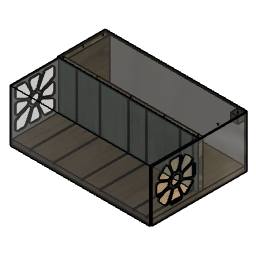
ionenantrieb v2 v2 (Autodesk Fusion 360 design; units mm, degrees)
Autodesk Fusion 360 part; units mm, degrees
sketch "Skizze1" plane through (0, 0, 0) normal (0, 0, 1) x (1, 0, 0)
  line L0 (0, 0) -> (300, 0)
  line L1 (300, 0) -> (300, 200)
  line L2 (300, 200) -> (0, 200)
  line L3 (0, 200) -> (0, 0)
  dimension "d1" = 300
  dimension "d2" = 200
  constraint horizontal L0
  constraint vertical L1
  constraint horizontal L2
  constraint vertical L3
  constraint coincident L0.start L3.end
  measures "d1" distance of L0.start L0.end
  measures "d2" distance of L0.start L2.end
extrude "Extrusion1" add sketch "Skizze1" along normal blind 10 makes body 1
sketch "Skizze2" plane through (0, 0, 10) normal (0, 0, 1) x (-1, 0, 0)
  line L0 (0, -200) -> (0, 0)
  line L1 (0, 0) -> (-300, 0)
  line L2 (-300, 0) -> (-300, -200)
  line L3 (-300, -200) -> (0, -200)
  line L4 (0, -100) -> (-300, -100)
  line L5 (-300, -100) -> (-300, -110)
  line L6 (-300, -110) -> (0, -110)
  line L7 (0, -110) -> (0, -100)
  constraint horizontal L4
  constraint vertical L5
  constraint horizontal L6
  constraint vertical L7
  constraint coincident L2 L5.end
  constraint midpoint L0 L4.start
extrude "Extrusion1'" add sketch "Skizze2" along normal blind 100 separate body contours L0 L2 L4 L5 L6 L7 makes body 2 in component "Component"
sketch "Skizze3" plane through (0, 200, 0) normal (0, 1, 0) x (-1, 0, 0)
  line L0 (-300, 0) -> (0, 0)
  line L1 (0, 0) -> (0, 10)
  line L2 (0, 10) -> (-300, 10)
  line L3 (-300, 10) -> (-300, 0)
  line L4 (-300, 0) -> (0, 0)
  line L5 (0, 0) -> (0, 110)
  line L6 (0, 110) -> (-300, 110)
  line L7 (-300, 110) -> (-300, 0)
  constraint horizontal L4
  constraint vertical L5
  constraint horizontal L6
  constraint vertical L7
  constraint coincident L0.start L3.end
extrude "Extrusion1''" add sketch "Skizze3" along normal blind 2.5 separate body makes body 3 in component "Component'"
sketch "Skizze4" plane through (0, 202.5, 0) normal (0, 1, 0) x (-1, 0, 0)
  line L0 (-300, 110) -> (-300, 0)
  line L1 (-300, 0) -> (0, 0)
  line L2 (0, 0) -> (0, 110)
  line L3 (0, 110) -> (-300, 110)
  circle A0 centre (-290, 5) radius 1
  circle A1 centre (-220, 5) radius 1
  circle A2 centre (-150, 5) radius 1
  circle A3 centre (-80, 5) radius 1
  circle A4 centre (-10, 5) radius 1
  dimension "d9" = 2
  dimension "d12" = 280
  dimension "d13" = 0
  measures "d9" diameter of A0
extrude "Extrusion2" cut sketch "Skizze4" against normal blind 2.5 contours A0 | A1 | A2 | A3 | A4 bodies 3 in component "Component'"
sketch "Skizze5" plane through (300, 0, 0) normal (1, 0, 0) x (0, 1, 0)
  line L0 (0, 0) -> (200, 0)
  line L1 (200, 0) -> (200, 10)
  line L2 (200, 10) -> (0, 10)
  line L3 (0, 10) -> (0, 0)
  line L4 (202.5, 0) -> (-1.5, 0)
  line L5 (-1.5, 0) -> (-1.5, 110)
  line L6 (-1.5, 110) -> (202.5, 110)
  line L7 (202.5, 110) -> (202.5, 0)
  dimension "d16" = 204
  constraint horizontal L4
  constraint vertical L5
  constraint horizontal L6
  constraint vertical L7
  measures "d16" distance of L4.start L4.end
extrude "Extrusion1'''" add sketch "Skizze5" along normal blind 2.5 separate body makes body 4 in component "Component''"
sketch "Skizze6" plane through (302.5, 0, 0) normal (1, 0, 0) x (0, 1, 0)
  line L0 (202.5, 110) -> (-1.5, 110)
  line L1 (-1.5, 110) -> (-1.5, 0)
  line L2 (-1.5, 0) -> (202.5, 0)
  line L3 (202.5, 0) -> (202.5, 110)
  circle A0 centre (10, 5) radius 1
  circle A1 centre (105, 5) radius 1
  line L4 (10, 5) -> (105, 5)
  circle A2 centre (57.5, 5) radius 1
  circle A3 centre (147.5, 5) radius 1
  circle A4 centre (190, 5) radius 1
  circle A5 centre (105, 52.5) radius 1
  circle A6 centre (105, 100) radius 1
  dimension "d19" = 2
  dimension "d20" = 2
  dimension "d21" = 2
  dimension "d24" = 85
  dimension "d25" = 0
  dimension "d28" = 0
  dimension "d29" = 95
  constraint coincident A0.centre L4.start
  constraint coincident A1.centre L4.end
  constraint midpoint L4 A2.centre
  measures "d19" diameter of A0
  measures "d20" diameter of A1
  measures "d21" diameter of A2
sketch "Skizze7" plane through (0, 0, 0) normal (-1, 0, 0) x (0, -1, 0)
  line L0 (-200, 0) -> (0, 0)
  line L1 (0, 0) -> (0, 10)
  line L2 (0, 10) -> (-200, 10)
  line L3 (-200, 10) -> (-200, 0)
  line L4 (-110, 110) -> (-200, 110)
  line L5 (-200, 110) -> (-200, 10)
  line L6 (-200, 10) -> (-110, 10)
  line L7 (-110, 10) -> (-110, 110)
  constraint horizontal L4
  constraint vertical L5
  constraint horizontal L6
  constraint vertical L7
  constraint coincident L2.end L3.start
extrude "Extrusion1''''" add sketch "Skizze7" against normal blind 10 separate body contours L2 L4 L5 L6 L7 makes body 5 in component "Component'''"
sketch "Skizze8" plane through (0, 0, 0) normal (-1, 0, 0) x (0, -1, 0)
  line L0 (-110, 10) -> (-100, 10)
  line L1 (-100, 10) -> (-100, 110)
  line L2 (-100, 110) -> (-110, 110)
  line L3 (-110, 110) -> (-110, 10)
  line L4 (-202.5, 0) -> (1.5, 0)
  line L5 (1.5, 0) -> (1.5, 110)
  line L6 (1.5, 110) -> (-202.5, 110)
  line L7 (-202.5, 110) -> (-202.5, 0)
  constraint horizontal L4
  constraint vertical L5
  constraint horizontal L6
  constraint vertical L7
extrude "Extrusion1'''''" add sketch "Skizze8" along normal blind 2.5 separate body makes body 6 in component "Component''''"
ref_plane "Arbeitsebene1" through (150, 100.5, 55) normal (1, 0, 0) x (0, 1, 0)
sketch "Skizze9" plane through (-2.5, 0, 0) normal (-1, 0, 0) x (0, -1, 0)
  line L0 (-202.5, 110) -> (-202.5, 0)
  line L1 (-202.5, 0) -> (1.5, 0)
  line L2 (1.5, 0) -> (1.5, 110)
  line L3 (1.5, 110) -> (-202.5, 110)
  circle A0 centre (-190, 5) radius 1
  circle A1 centre (-10, 5) radius 1
  circle A2 centre (-105, 5) radius 1
  circle A3 centre (-150, 5) radius 1
  circle A4 centre (-57.5, 5) radius 1
  circle A5 centre (-105, 52.5) radius 1
  circle A6 centre (-105, 100) radius 1
  dimension "d34" = 2
  dimension "d35" = 2
  dimension "d36" = 2
  dimension "d37" = 2
  dimension "d38" = 2
  dimension "d41" = 0
  dimension "d42" = 95
  measures "d34" diameter of A0
  measures "d35" diameter of A1
  measures "d36" diameter of A2
  measures "d37" diameter of A3
  measures "d38" diameter of A4
extrude "Extrusion2'" cut sketch "Skizze9" against normal blind 2.5 contours A0 | A1 | A2 | A3 | A4 | A5 | A6 bodies 6 in component "Component''''"
sketch "Skizze10" plane through (0, 0, 110) normal (0, 0, 1) x (-1, 0, 0)
  line L0 (0, -110) -> (0, -100)
  line L1 (0, -100) -> (-300, -100)
  line L2 (-300, -100) -> (-300, -110)
  line L3 (-300, -110) -> (0, -110)
  line L4 (-302.5, -202.5) -> (2.5, -202.5)
  line L5 (2.5, -202.5) -> (2.5, -100)
  line L6 (2.5, -100) -> (-302.5, -100)
  line L7 (-302.5, -100) -> (-302.5, -202.5)
  constraint horizontal L4
  constraint vertical L5
  constraint horizontal L6
  constraint vertical L7
extrude "Extrusion1''''''" add sketch "Skizze10" along normal blind 2.5 separate body makes body 7 in component "Component'''''"
sketch "Skizze11" plane through (0, 0, 112.5) normal (0, 0, 1) x (-1, 0, 0)
  line L0 (-302.5, -100) -> (-302.5, -202.5)
  line L1 (-302.5, -202.5) -> (2.5, -202.5)
  line L2 (2.5, -202.5) -> (2.5, -100)
  line L3 (2.5, -100) -> (-302.5, -100)
  circle A0 centre (-295, -105) radius 1
  circle A1 centre (-222.5, -105) radius 1
  circle A2 centre (-150, -105) radius 1
  circle A3 centre (-77.5, -105) radius 1
  circle A4 centre (-5, -105) radius 1
  circle A5 centre (-5, -190) radius 1
  line L4 (-5, -190) -> (-5, -105)
  circle A6 centre (-5, -147.5) radius 1
  line L5 (-150, -105) -> (-150, -112.2245)
  circle A7 centre (-295, -147.5) radius 1
  circle A8 centre (-295, -190) radius 1
  point P0 (-295, -190)
  dimension "d47" = 2
  dimension "d50" = 290
  dimension "d51" = 0
  dimension "d52" = 2
  dimension "d53" = 2
  constraint coincident A5.centre L4.start
  constraint coincident A4.centre L4.end
  constraint perpendicular L3 L4
  constraint midpoint L4 A6.centre
  constraint coincident A2.centre L5.start
  constraint vertical L5
  constraint symmetric A5 L5 A8
  constraint symmetric A5.centre L5 P0
  constraint symmetric A6 L5 A7
  measures "d47" diameter of A0
  measures "d52" diameter of A5
  measures "d53" diameter of A6
extrude "Extrusion2''" cut sketch "Skizze11" against normal blind 2.5 contours A0 | A1 | A2 | A3 | A4 | A5 | L4 A6 | L4 A6 | A7 | A8 bodies 7 in component "Component'''''"
sketch "Skizze12" plane through (0, 200, 0) normal (0, -1, 0) x (1, 0, 0)
  circle A0 centre (80, 5) radius 1
  circle A1 centre (290, 5) radius 1
  circle A2 centre (220, 5) radius 1
  circle A3 centre (150, 5) radius 1
  circle A4 centre (10, 5) radius 1
  line L0 (300, 0) -> (300, 110)
  line L1 (300, 110) -> (0, 110)
  line L2 (0, 110) -> (0, 0)
  line L3 (0, 0) -> (300, 0)
  line L4 (300, 110) -> (285, 110)
  line L5 (285, 110) -> (285, 95)
  line L6 (285, 95) -> (300, 95)
  line L7 (300, 95) -> (300, 110)
  constraint horizontal L4
  constraint vertical L5
  constraint horizontal L6
  constraint vertical L7
  constraint coincident L0.end L1.start
extrude "Extrusion1'''''''" add sketch "Skizze12" along normal blind 15 separate body contours L0 L1 L4 L5 L6 L7 makes body 8 in component "Component''''''"
sketch "Skizze13" plane through (302.5, 0, 0) normal (1, 0, 0) x (0, 1, 0)
  line L0 (202.5, 110) -> (-1.5, 110)
  line L1 (-1.5, 110) -> (-1.5, 0)
  line L2 (-1.5, 0) -> (202.5, 0)
  line L3 (202.5, 0) -> (202.5, 110)
  line L4 (100, 10) -> (0, 10)
  line L5 (0, 10) -> (0, 110)
  line L6 (0, 110) -> (100, 110)
  line L7 (100, 110) -> (100, 10)
  circle A0 centre (50, 60) radius 10
  line L8 (92, 18) -> (8, 18)
  line L9 (8, 18) -> (8, 102)
  line L10 (41.854, 102) -> (58.146, 102)
  line L11 (92, 102) -> (92, 18)
  arc A1 (51.1575, 73.9521) -> (48.8425, 73.9521) centre (50, 60) ccw
  line L12 (50, 60) -> (50, 70)
  line L13 (50, 60) -> (46.5798, 69.3969)
  line L14 (43.7307, 77.2249) -> (37.1555, 95.2899)
  line L15 (50, 60) -> (53.4202, 69.3969)
  line L16 (56.2693, 77.2249) -> (62.8445, 95.2899)
  arc A2 (41.854, 102) -> (37.1555, 95.2899) centre (41.854, 97) ccw
  arc A3 (62.8445, 95.2899) -> (58.146, 102) centre (58.146, 97) ccw
  arc A4 (43.7307, 77.2249) -> (48.8425, 73.9521) centre (48.4291, 78.935) ccw
  arc A5 (51.1575, 73.9521) -> (56.2693, 77.2249) centre (51.5709, 78.935) ccw
  line L17 (14.5414, 83.9384) -> (26.0616, 95.4586)
  arc A6 (33.3871, 67.7467) -> (39.3159, 69.0471) centre (35.5002, 72.2783) ccw
  line L18 (42.2533, 76.6129) -> (34.1287, 94.0361)
  arc A7 (14.5414, 83.9384) -> (15.9639, 75.8713) centre (18.077, 80.4029) ccw
  arc A8 (40.9529, 70.6841) -> (39.3159, 69.0471) centre (50, 60) ccw
  line L19 (33.3871, 67.7467) -> (15.9639, 75.8713)
  arc A9 (40.9529, 70.6841) -> (42.2533, 76.6129) centre (37.7217, 74.4998) ccw
  arc A10 (34.1287, 94.0361) -> (26.0616, 95.4586) centre (29.5971, 91.923) ccw
  line L20 (8, 51.854) -> (8, 68.146)
  arc A11 (32.7752, 53.7307) -> (36.0479, 58.8425) centre (31.065, 58.4291) ccw
  line L21 (32.7752, 66.2693) -> (14.7101, 72.8445)
  arc A12 (8, 51.854) -> (14.7101, 47.1555) centre (13, 51.854) ccw
  arc A13 (36.0479, 61.1575) -> (36.0479, 58.8425) centre (50, 60) ccw
  line L22 (32.7752, 53.7307) -> (14.7101, 47.1555)
  arc A14 (36.0479, 61.1575) -> (32.7752, 66.2693) centre (31.065, 61.5709) ccw
  arc A15 (14.7101, 72.8445) -> (8, 68.146) centre (13, 68.146) ccw
  line L23 (26.0616, 24.5414) -> (14.5414, 36.0616)
  arc A16 (42.2533, 43.3871) -> (40.9529, 49.3159) centre (37.7217, 45.5002) ccw
  line L24 (33.3871, 52.2533) -> (15.9639, 44.1287)
  arc A17 (26.0616, 24.5414) -> (34.1287, 25.9639) centre (29.5971, 28.077) ccw
  arc A18 (39.3159, 50.9529) -> (40.9529, 49.3159) centre (50, 60) ccw
  line L25 (42.2533, 43.3871) -> (34.1287, 25.9639)
  arc A19 (39.3159, 50.9529) -> (33.3871, 52.2533) centre (35.5002, 47.7217) ccw
  arc A20 (15.9639, 44.1287) -> (14.5414, 36.0616) centre (18.077, 39.5971) ccw
  line L26 (58.146, 18) -> (41.854, 18)
  arc A21 (56.2693, 42.7751) -> (51.1575, 46.0479) centre (51.5709, 41.065) ccw
  line L27 (43.7307, 42.7751) -> (37.1555, 24.7101)
  arc A22 (58.146, 18) -> (62.8445, 24.7101) centre (58.146, 23) ccw
  arc A23 (48.8425, 46.0479) -> (51.1575, 46.0479) centre (50, 60) ccw
  line L28 (56.2693, 42.7751) -> (62.8445, 24.7101)
  arc A24 (48.8425, 46.0479) -> (43.7307, 42.7751) centre (48.4291, 41.065) ccw
  arc A25 (37.1555, 24.7101) -> (41.854, 18) centre (41.854, 23) ccw
  line L29 (85.4586, 36.0616) -> (73.9384, 24.5414)
  arc A26 (66.6129, 52.2533) -> (60.6841, 50.9529) centre (64.4998, 47.7217) ccw
  line L30 (57.7467, 43.3871) -> (65.8713, 25.9639)
  arc A27 (85.4586, 36.0616) -> (84.0361, 44.1287) centre (81.9231, 39.5971) ccw
  arc A28 (59.0471, 49.3159) -> (60.6841, 50.9529) centre (50, 60) ccw
  line L31 (66.6129, 52.2533) -> (84.0361, 44.1287)
  arc A29 (59.0471, 49.3159) -> (57.7467, 43.3871) centre (62.2783, 45.5002) ccw
  arc A30 (65.8713, 25.9639) -> (73.9384, 24.5414) centre (70.4029, 28.077) ccw
  line L32 (92, 68.146) -> (92, 51.854)
  arc A31 (67.2249, 66.2693) -> (63.9521, 61.1575) centre (68.935, 61.5709) ccw
  line L33 (67.2249, 53.7307) -> (85.2899, 47.1555)
  arc A32 (92, 68.146) -> (85.2899, 72.8445) centre (87, 68.146) ccw
  arc A33 (63.9521, 58.8425) -> (63.9521, 61.1575) centre (50, 60) ccw
  line L34 (67.2249, 66.2693) -> (85.2899, 72.8445)
  arc A34 (63.9521, 58.8425) -> (67.2249, 53.7307) centre (68.935, 58.4291) ccw
  arc A35 (85.2899, 47.1555) -> (92, 51.854) centre (87, 51.854) ccw
  line L35 (73.9384, 95.4586) -> (85.4586, 83.9384)
  arc A36 (57.7467, 76.6129) -> (59.0471, 70.6841) centre (62.2783, 74.4998) ccw
  line L36 (66.6129, 67.7467) -> (84.0361, 75.8713)
  arc A37 (73.9384, 95.4586) -> (65.8713, 94.0361) centre (70.4029, 91.923) ccw
  arc A38 (60.6841, 69.0471) -> (59.0471, 70.6841) centre (50, 60) ccw
  line L37 (57.7467, 76.6129) -> (65.8713, 94.0361)
  arc A39 (60.6841, 69.0471) -> (66.6129, 67.7467) centre (64.4998, 72.2783) ccw
  arc A40 (84.0361, 75.8713) -> (85.4586, 83.9384) centre (81.9231, 80.4029) ccw
  dimension "d58" = 20
  dimension "d61" = 20
  dimension "d62" = 20
  dimension "d63" = 5
  dimension "d64" = 5
  dimension "d66" = 360
  constraint horizontal L4
  constraint vertical L5
  constraint horizontal L6
  constraint vertical L7
  constraint coincident L0 L5.end
  constraint coincident A0.centre A1.centre
  constraint perpendicular L10 L12
  constraint concentric A0 A1
  constraint coincident A0 L12.end
  constraint coincident A0 L13.end
  constraint collinear L13 L14
  constraint coincident A0 L15.end
  constraint collinear L15 L16
  constraint parallel L4 L8
  constraint parallel L5 L9
  constraint parallel L6 L10
  constraint parallel L7 L11
  constraint tangent L14 A2
  constraint tangent L10 A2
  constraint tangent L16 A3
  constraint tangent L10 A3
  constraint equal A2 A3
  constraint tangent L14 A4
  constraint tangent A1 A4
  constraint tangent L16 A5
  constraint tangent A1 A5
  constraint equal A4 A5
  measures "d58" diameter of A0
  measures "d61" angle of L12 L15
  measures "d62" angle of L12 L13
  measures "d63" radius of A2
  measures "d64" radius of A4
extrude "Extrusion2'''" cut sketch "Skizze13" against normal blind 5 contours A0 L13 L15 | A0 L12 L15 | A0 L12 L13 | L8 L26 A21 L27 A22 A23 L28 A24 A25 | L9 L20 A11 L21 A12 A13 L22 A14 A15 | L10 A1 L14 L16 A2 A3 A4 A5 | L11 L32 A31 L33 A32 A33 L34 A34 A35 | L17 A6 L18 A7 A8 L19 A9 A10 | L23 A16 L24 A17 A18 L25 A19 A20 | L29 A26 L30 A27 A28 L31 A29 A30 | L35 A36 L36 A37 A38 L37 A39 A40 bodies 4 in component "Component''"
sketch "Skizze14" plane through (-2.5, 0, 0) normal (-1, 0, 0) x (0, -1, 0)
  circle A0 centre (-105, 100) radius 1
  circle A1 centre (-57.5, 5) radius 1
  circle A2 centre (-105, 5) radius 1
  circle A3 centre (-10, 5) radius 1
  circle A4 centre (-190, 5) radius 1
  circle A5 centre (-105, 52.5) radius 1
  circle A6 centre (-150, 5) radius 1
  line L0 (-202.5, 110) -> (-202.5, 0)
  line L1 (-202.5, 0) -> (1.5, 0)
  line L2 (1.5, 0) -> (1.5, 110)
  line L3 (1.5, 110) -> (-202.5, 110)
  line L4 (-100, 110) -> (0, 110)
  line L5 (0, 110) -> (0, 10)
  line L6 (0, 10) -> (-100, 10)
  line L7 (-100, 10) -> (-100, 110)
  circle A7 centre (-50, 60) radius 10
  line L8 (-50, 70) -> (-50, 74)
  line L9 (-92, 60) -> (-92, 67.452)
  line L10 (-92, 83.6091) -> (-92, 97)
  line L11 (-66.4752, 68.0355) -> (-89.1919, 79.1151)
  line L12 (-67.3316, 65.9678) -> (-85.3722, 72.1796)
  line L13 (-33.5248, 68.0355) -> (-10.8081, 79.1151)
  line L14 (-32.6684, 65.9678) -> (-14.6278, 72.1796)
  line L15 (-44.0322, 77.3316) -> (-37.8204, 95.3722)
  line L16 (-41.9645, 76.4752) -> (-30.8849, 99.1919)
  line L17 (-55.9678, 77.3316) -> (-62.1796, 95.3722)
  line L18 (-58.0355, 76.4752) -> (-69.1151, 99.1919)
  line L19 (-87, 102) -> (-73.6091, 102)
  line L20 (-57.452, 102) -> (-42.548, 102)
  line L21 (-26.3909, 102) -> (-13, 102)
  line L22 (-8, 97) -> (-8, 83.6091)
  line L23 (-8, 67.452) -> (-8, 60)
  arc A8 (-87, 102) -> (-92, 97) centre (-87, 97) ccw
  arc A9 (-57.452, 102) -> (-62.1796, 95.3722) centre (-57.452, 97) ccw
  arc A10 (-37.8204, 95.3722) -> (-42.548, 102) centre (-42.548, 97) ccw
  arc A11 (-8, 97) -> (-13, 102) centre (-13, 97) ccw
  arc A12 (-69.1151, 99.1919) -> (-73.6091, 102) centre (-73.6091, 97) ccw
  arc A13 (-92, 83.6091) -> (-89.1919, 79.1151) centre (-87, 83.6091) ccw
  arc A14 (-26.3909, 102) -> (-30.8849, 99.1919) centre (-26.3909, 97) ccw
  arc A15 (-10.8081, 79.1151) -> (-8, 83.6091) centre (-13, 83.6091) ccw
  arc A16 (-8, 67.452) -> (-14.6278, 72.1796) centre (-13, 67.452) ccw
  arc A17 (-85.3722, 72.1796) -> (-92, 67.452) centre (-87, 67.452) ccw
  arc A18 (-59.2322, 70.5245) -> (-60.5245, 69.2322) centre (-50, 60) ccw
  arc A19 (-49.0862, 73.9701) -> (-50.9138, 73.9701) centre (-50, 60) ccw
  arc A20 (-63.9701, 60.9138) -> (-36.0299, 60.9138) centre (-50, 60) ccw
  arc A21 (-39.4755, 69.2322) -> (-40.7678, 70.5245) centre (-50, 60) ccw
  arc A22 (-66.4752, 68.0355) -> (-60.5245, 69.2322) centre (-64.2833, 72.5294) ccw
  arc A23 (-59.2322, 70.5245) -> (-58.0355, 76.4752) centre (-62.5294, 74.2833) ccw
  arc A24 (-55.9678, 77.3316) -> (-50.9138, 73.9701) centre (-51.2402, 78.9595) ccw
  arc A25 (-49.0862, 73.9701) -> (-44.0322, 77.3316) centre (-48.7598, 78.9595) ccw
  arc A26 (-41.9645, 76.4752) -> (-40.7678, 70.5245) centre (-37.4706, 74.2833) ccw
  arc A27 (-39.4755, 69.2322) -> (-33.5248, 68.0355) centre (-35.7167, 72.5294) ccw
  arc A28 (-63.9701, 60.9138) -> (-67.3316, 65.9678) centre (-68.9595, 61.2402) ccw
  arc A29 (-32.6684, 65.9678) -> (-36.0299, 60.9138) centre (-31.0405, 61.2402) ccw
  line L24 (-92, 60) -> (-85, 60)
  arc A30 (-92, 23) -> (-87, 18) centre (-87, 23) ccw
  arc A31 (-62.1796, 24.6278) -> (-57.452, 18) centre (-57.452, 23) ccw
  line L25 (-66.4752, 51.9645) -> (-89.1919, 40.8849)
  line L26 (-92, 36.3909) -> (-92, 23)
  arc A32 (-73.6091, 18) -> (-69.1151, 20.8081) centre (-73.6091, 23) ccw
  arc A33 (-60.5245, 50.7678) -> (-59.2322, 49.4755) centre (-50, 60) ccw
  arc A34 (-58.0355, 43.5248) -> (-59.2322, 49.4755) centre (-62.5294, 45.7167) ccw
  line L27 (-55.9678, 42.6684) -> (-62.1796, 24.6278)
  line L28 (-50, 50) -> (-50, 46)
  arc A35 (-92, 52.548) -> (-85.3722, 47.8204) centre (-87, 52.548) ccw
  line L29 (-87, 18) -> (-73.6091, 18)
  arc A36 (-50.9138, 46.0299) -> (-55.9678, 42.6684) centre (-51.2402, 41.0405) ccw
  line L30 (-67.3316, 54.0322) -> (-85.3722, 47.8204)
  arc A37 (-50.9138, 46.0299) -> (-49.0862, 46.0299) centre (-50, 60) ccw
  arc A38 (-89.1919, 40.8849) -> (-92, 36.3909) centre (-87, 36.3909) ccw
  line L31 (-58.0355, 43.5248) -> (-69.1151, 20.8081)
  arc A39 (-67.3316, 54.0322) -> (-63.9701, 59.0862) centre (-68.9595, 58.7598) ccw
  line L32 (-92, 60) -> (-92, 52.548)
  arc A40 (-33.5248, 51.9645) -> (-39.4755, 50.7678) centre (-35.7167, 47.4706) ccw
  arc A41 (-44.0322, 42.6684) -> (-49.0862, 46.0299) centre (-48.7598, 41.0405) ccw
  arc A42 (-14.6278, 47.8204) -> (-8, 52.548) centre (-13, 52.548) ccw
  line L33 (-32.6684, 54.0322) -> (-14.6278, 47.8204)
  line L34 (-26.3909, 18) -> (-13, 18)
  line L35 (-41.9645, 43.5248) -> (-30.8849, 20.8081)
  arc A43 (-40.7678, 49.4755) -> (-39.4755, 50.7678) centre (-50, 60) ccw
  line L36 (-57.452, 18) -> (-42.548, 18)
  line L37 (-8, 52.548) -> (-8, 60)
  arc A44 (-13, 18) -> (-8, 23) centre (-13, 23) ccw
  line L38 (-44.0322, 42.6684) -> (-37.8204, 24.6278)
  arc A45 (-36.0299, 59.0862) -> (-32.6684, 54.0322) centre (-31.0405, 58.7598) ccw
  arc A46 (-40.7678, 49.4755) -> (-41.9645, 43.5248) centre (-37.4706, 45.7167) ccw
  line L39 (-33.5248, 51.9645) -> (-10.8081, 40.8849)
  arc A47 (-42.548, 18) -> (-37.8204, 24.6278) centre (-42.548, 23) ccw
  line L40 (-8, 23) -> (-8, 36.3909)
  arc A48 (-8, 36.3909) -> (-10.8081, 40.8849) centre (-13, 36.3909) ccw
  arc A49 (-30.8849, 20.8081) -> (-26.3909, 18) centre (-26.3909, 23) ccw
  arc A50 (-60.5245, 50.7678) -> (-66.4752, 51.9645) centre (-64.2833, 47.4706) ccw
  point P0 (-50, 60)
  point P1 (-50, 60)
  dimension "d70" = 20
  dimension "d80" = 5
  dimension "d81" = 5
  dimension "d82" = 5
  dimension "d83" = 5
  constraint horizontal L4
  constraint vertical L5
  constraint horizontal L6
  constraint vertical L7
  constraint coincident L3 L4.start
  constraint parallel L7 L9
  constraint parallel L4 L19
  constraint parallel L5 L22
  constraint collinear L9 L10
  constraint coincident A7 L8.start
  constraint collinear L19 L20
  constraint collinear L20 L21
  constraint coincident L8.end A20
  constraint collinear L22 L23
  constraint coincident L23.end L22
  constraint tangent L19 A8
  constraint tangent L10 A8
  constraint tangent L20 A9
  constraint tangent L17 A9
  constraint equal A8 A9
  constraint tangent L15 A10
  constraint tangent L20 A10
  constraint equal A8 A10
  constraint tangent L21 A11
  constraint tangent L22 A11
  constraint equal A8 A11
  constraint tangent L18 A12
  constraint tangent L19 A12
  constraint equal A8 A12
  constraint tangent L11 A13
  constraint tangent L10 A13
  constraint equal A8 A13
  constraint tangent L16 A14
  constraint tangent L21 A14
  constraint equal A8 A14
  constraint tangent L13 A15
  constraint tangent L22 A15
  constraint equal A8 A15
  constraint tangent L14 A16
  constraint tangent L23 A16
  constraint equal A8 A16
  constraint tangent L12 A17
  constraint tangent L9 A17
  constraint equal A8 A17
  constraint concentric A7 A20
  constraint concentric A18 A20
  constraint concentric A19 A20
  constraint concentric A20 A21
  constraint tangent A18 A22
  constraint tangent L11 A22
  constraint tangent L18 A23
  constraint tangent A18 A23
  constraint equal A22 A23
  constraint tangent L17 A24
  constraint tangent A19 A24
  constraint equal A22 A24
  constraint tangent A19 A25
  constraint tangent L15 A25
  constraint equal A22 A25
  constraint tangent A21 A26
  constraint tangent L16 A26
  constraint equal A22 A26
  constraint tangent L13 A27
  constraint tangent A21 A27
  constraint equal A22 A27
  constraint tangent A20 A28
  constraint tangent L12 A28
  constraint tangent L14 A29
  constraint tangent A20 A29
  constraint perpendicular L9 L24
  constraint symmetric P1 L24 P0
  constraint symmetric L9.start L24 L32.start
  constraint symmetric L23.end L24 L37.end
  constraint symmetric L8.start L24 L28.start
  constraint symmetric L8.end L24 L28.end
  constraint symmetric L19.start L24 A30.end
  constraint symmetric L10.end L24 A30.start
  constraint symmetric A8 L24 A30
  constraint symmetric L20.start L24 A31.end
  constraint symmetric L17.end L24 A31.start
  constraint symmetric A9 L24 A31
  constraint symmetric L15.end L24 L38.end
  constraint symmetric L20.end L24 L36.end
  constraint symmetric A10 L24 A47
  constraint symmetric L21.end L24 L34.end
  constraint symmetric L22.start L24 A44.end
  constraint symmetric A11 L24 A44
  constraint symmetric L18.end L24 A32.end
  constraint symmetric L19.end L24 A32.start
  constraint symmetric A12 L24 A32
  constraint symmetric L11.end L24 L25.end
  constraint symmetric L10.start L24 L26.start
  constraint symmetric A13 L24 A38
  constraint symmetric L16.end L24 L35.end
  constraint symmetric L21.start L24 L34.start
  constraint symmetric A14 L24 A49
  constraint symmetric L13.end L24 L39.end
  constraint symmetric L22.end L24 L40.end
  constraint symmetric A15 L24 A48
  constraint symmetric L14.end L24 A42.start
  constraint symmetric L23.start L24 A42.end
  constraint symmetric A16 L24 A42
  constraint symmetric L12.end L24 A35.end
  constraint symmetric L9.end L24 A35.start
  constraint symmetric A17 L24 A35
  constraint symmetric A18 L24 A33
  constraint symmetric A19 L24 A37
  constraint symmetric A21 L24 A43
  constraint symmetric L11.start L24 L25.start
  constraint symmetric A18.end L24 A33.start
  constraint symmetric A22 L24 A50
  constraint symmetric L18.start L24 A34.start
  constraint symmetric A18.start L24 A33.end
  constraint symmetric A23 L24 A34
  constraint symmetric L17.start L24 L27.start
  constraint symmetric A19.end L24 A36.start
  constraint symmetric A24 L24 A36
  constraint symmetric L15.start L24 A41.start
  constraint symmetric A19.start L24 A37.end
  constraint symmetric A25 L24 A41
  constraint symmetric L16.start L24 L35.start
  constraint symmetric A21.end L24 A43.start
  constraint symmetric A26 L24 A46
  constraint symmetric L13.start L24 A40.start
  constraint symmetric A21.start L24 A40.end
  constraint symmetric A27 L24 A40
  constraint symmetric L12.start L24 L30.start
  constraint symmetric A20.start L24 A39.end
  constraint symmetric A28 L24 A39
  constraint symmetric L14.start L24 L33.start
  constraint symmetric A20.end L24 A45.start
  constraint symmetric A29 L24 A45
  measures "d70" diameter of A7
  measures "d80" radius of A8
  measures "d81" radius of A22
  measures "d82" radius of A28
  measures "d83" radius of A29
extrude "Extrusion3" cut sketch "Skizze14" against normal blind 2.5 contours A7 | L9 L12 A17 A20 A28 A35 L30 A39 L32 | L10 L11 L18 L19 A8 A12 A13 A18 A22 A23 | L13 L16 L21 L22 A11 A14 A15 A21 A26 A27 | L14 L23 A16 A20 A29 A42 L33 L37 A45 | L15 L17 L20 A9 A10 A19 A24 A25 | A20 A30 L25 L26 A32 A33 A34 L29 A38 L31 A50 | A20 A31 L27 A36 A37 A41 L36 L38 A47 | A20 A40 L34 L35 A43 A44 A46 L39 L40 A48 A49 bodies 6 in component "Component''''"
sketch "Skizze15" plane through (0, 0, 10) normal (0, 0, 1) x (-1, 0, 0)
  line L0 (0, -200) -> (0, 0)
  line L1 (0, 0) -> (-300, 0)
  line L2 (-300, 0) -> (-300, -200)
  line L3 (-300, -200) -> (0, -200)
  line L4 (-290, 0) -> (-287.4, 0)
  line L5 (-287.4, 0) -> (-287.4, -100)
  line L6 (-287.4, -100) -> (-290, -100)
  line L7 (-290, -100) -> (-290, 0)
  line L8 (-259.8, 0) -> (-259.8, -100)
  line L9 (-262.4, -100) -> (-262.4, 0)
  line L10 (-259.8, -100) -> (-262.4, -100)
  line L11 (-262.4, 0) -> (-259.8, 0)
  line L12 (-187.4, 0) -> (-187.4, -100)
  line L13 (-190, -100) -> (-190, 0)
  line L14 (-190, 0) -> (-187.4, 0)
  line L15 (-187.4, -100) -> (-190, -100)
  line L16 (-148.9, 0) -> (-148.9, -100)
  line L17 (-151.5, -100) -> (-151.5, 0)
  line L18 (-151.5, 0) -> (-148.9, 0)
  line L19 (-148.9, -100) -> (-151.5, -100)
  line L20 (-87.4, 0) -> (-87.4, -100)
  line L21 (-90, -100) -> (-90, 0)
  line L22 (-87.4, -100) -> (-90, -100)
  line L23 (-90, 0) -> (-87.4, 0)
  line L24 (-40, -100) -> (-40, 0)
  line L25 (-37.4, 0) -> (-37.4, -100)
  line L26 (-40, 0) -> (-37.4, 0)
  line L27 (-37.4, -100) -> (-40, -100)
  dimension "d86" = 100
  dimension "d87" = 2.6
  dimension "d90" = 27.6
  dimension "d91" = 0
  dimension "d94" = 72.4
  dimension "d95" = 0
  dimension "d98" = 38.5
  dimension "d99" = 0
  dimension "d102" = 100
  dimension "d103" = 0
  dimension "d106" = 50
  dimension "d107" = 0
  constraint horizontal L4
  constraint vertical L5
  constraint horizontal L6
  constraint vertical L7
  constraint coincident L1 L4.start
  measures "d86" distance of L4.start L6.end
  measures "d87" distance of L4.start L4.end
extrude "Extrusion2''''" cut sketch "Skizze15" against normal blind 3 contours L1 L24 L25 L26 L27 | L1 L4 L5 L6 L7 | L1 L20 L21 L22 L23 | L1 L8 L9 L10 L11 | L1 L16 L17 L18 L19 | L1 L12 L13 L14 L15 bodies 1
sketch "Skizze16" plane through (0, 100, 0) normal (0, -1, 0) x (1, 0, 0)
  line L0 (0, 10) -> (300, 10)
  line L1 (300, 10) -> (300, 110)
  line L2 (300, 110) -> (0, 110)
  line L3 (0, 110) -> (0, 10)
sketch "Skizze17" plane through (0, 0, 0) normal (0, -1, 0) x (1, 0, 0)
  line L0 (187.4, 7) -> (187.4, 10)
  line L1 (187.4, 10) -> (151.5, 10)
  line L2 (151.5, 10) -> (151.5, 7)
  line L3 (151.5, 7) -> (148.9, 7)
  line L4 (148.9, 7) -> (148.9, 10)
  line L5 (148.9, 10) -> (90, 10)
  line L6 (90, 10) -> (90, 7)
  line L7 (90, 7) -> (87.4, 7)
  line L8 (87.4, 7) -> (87.4, 10)
  line L9 (87.4, 10) -> (40, 10)
  line L10 (40, 10) -> (40, 7)
  line L11 (40, 7) -> (37.4, 7)
  line L12 (37.4, 7) -> (37.4, 10)
  line L13 (37.4, 10) -> (0, 10)
  line L14 (0, 10) -> (0, 0)
  line L15 (0, 0) -> (300, 0)
  line L16 (300, 0) -> (300, 10)
  line L17 (300, 10) -> (290, 10)
  line L18 (290, 10) -> (290, 7)
  line L19 (290, 7) -> (287.4, 7)
  line L20 (287.4, 7) -> (287.4, 10)
  line L21 (287.4, 10) -> (262.4, 10)
  line L22 (262.4, 10) -> (262.4, 7)
  line L23 (262.4, 7) -> (259.8, 7)
  line L24 (259.8, 7) -> (259.8, 10)
  line L25 (259.8, 10) -> (190, 10)
  line L26 (190, 10) -> (190, 7)
  line L27 (190, 7) -> (187.4, 7)
  line L28 (0, 0) -> (300, 0)
  line L29 (300, 0) -> (300, 10)
  line L30 (300, 10) -> (290, 10)
  line L31 (290, 10) -> (290, 7)
  line L32 (290, 7) -> (287.4, 7)
  line L33 (287.4, 7) -> (287.4, 10)
  line L34 (287.4, 10) -> (262.4, 10)
  line L35 (262.4, 10) -> (262.4, 7)
  line L36 (262.4, 7) -> (259.8, 7)
  line L37 (259.8, 7) -> (259.8, 10)
  line L38 (259.8, 10) -> (190, 10)
  line L39 (190, 10) -> (190, 7)
  line L40 (190, 7) -> (187.4, 7)
  line L41 (187.4, 7) -> (187.4, 10)
  line L42 (187.4, 10) -> (151.5, 10)
  line L43 (151.5, 10) -> (151.5, 7)
  line L44 (151.5, 7) -> (148.9, 7)
  line L45 (148.9, 7) -> (148.9, 10)
  line L46 (148.9, 10) -> (90, 10)
  line L47 (90, 10) -> (90, 7)
  line L48 (90, 7) -> (87.4, 7)
  line L49 (87.4, 7) -> (87.4, 10)
  line L50 (87.4, 10) -> (40, 10)
  line L51 (40, 10) -> (40, 7)
  line L52 (40, 7) -> (37.4, 7)
  line L53 (37.4, 7) -> (37.4, 10)
  line L54 (37.4, 10) -> (0, 10)
  line L55 (0, 10) -> (0, 0)
  dimension "d110" = 0
  measures "d110" distance of L15
sketch "Skizze18" plane through (0, 100, 0) normal (0, -1, 0) x (1, 0, 0)
  line L0 (40, 10) -> (37.4, 10)
  line L1 (37.4, 10) -> (37.4, 110)
  line L2 (37.4, 110) -> (40, 110)
  line L3 (40, 110) -> (40, 10)
  line L4 (90, 10) -> (87.4, 10)
  line L5 (87.4, 10) -> (87.4, 110)
  line L6 (90, 110) -> (90, 10)
  line L7 (87.4, 110) -> (90, 110)
  line L8 (190, 10) -> (187.4, 10)
  line L9 (187.4, 110) -> (190, 110)
  line L10 (187.4, 10) -> (187.4, 110)
  line L11 (190, 110) -> (190, 10)
  line L12 (290, 10) -> (287.4, 10)
  line L13 (287.4, 110) -> (290, 110)
  line L14 (287.4, 10) -> (287.4, 110)
  line L15 (290, 110) -> (290, 10)
  line L16 (148.9, 110) -> (151.5, 110)
  line L17 (151.5, 110) -> (151.5, 10)
  line L18 (148.9, 10) -> (148.9, 110)
  line L19 (151.5, 10) -> (148.9, 10)
  line L20 (262.4, 10) -> (259.8, 10)
  line L21 (259.8, 10) -> (259.8, 110)
  line L22 (259.8, 110) -> (262.4, 110)
  line L23 (262.4, 110) -> (262.4, 10)
  dimension "d111" = 2.6
  dimension "d112" = 100
  dimension "d113" = 2.6
  dimension "d114" = 100
  dimension "d117" = 200
  dimension "d118" = 0
  dimension "d119" = 2.6
  dimension "d120" = 100
  dimension "d121" = 2.6
  dimension "d122" = 100
  constraint horizontal L0
  constraint vertical L1
  constraint horizontal L2
  constraint vertical L3
  constraint horizontal L4
  constraint vertical L5
  constraint horizontal L7
  constraint vertical L6
  constraint horizontal L19
  constraint vertical L18
  constraint horizontal L16
  constraint vertical L17
  constraint horizontal L20
  constraint vertical L21
  constraint horizontal L22
  constraint vertical L23
  measures "d111" distance of L0.start L0.end
  measures "d112" distance of L0.start L2.end
  measures "d113" distance of L4.start L4.end
  measures "d114" distance of L4.start L6.start
  measures "d119" distance of L18.start L17.end
  measures "d120" distance of L16.end L17.end
  measures "d121" distance of L20.start L20.end
  measures "d122" distance of L20.start L22.end
extrude "Extrusion2'''''" cut sketch "Skizze18" against normal blind 2.5 bodies 2 in component "Component"
sketch "Skizze19" plane through (0, 0, 110) normal (0, 0, 1) x (-1, 0, 0)
  line L0 (-300, -202.5) -> (-300, 1.5)
  line L1 (-300, 1.5) -> (-302.5, 1.5)
  line L2 (-302.5, 1.5) -> (-302.5, -202.5)
  line L3 (-302.5, -202.5) -> (-300, -202.5)
  line L4 (-300, -100.5) -> (0, -100.5)
  line L5 (0, -100.5) -> (0, 2)
  line L6 (0, 2) -> (-300, 2)
  line L7 (-300, 2) -> (-300, -100.5)
  dimension "d125" = 102.5
  constraint horizontal L4
  constraint vertical L5
  constraint horizontal L6
  constraint vertical L7
  constraint midpoint L0 L4.start
  measures "d125" distance of L4.end L5.end
extrude "Extrusion1''''''''" add sketch "Skizze19" along normal blind 2.5 separate body contours L0 L4 L5 L6 L7 makes body 9 in component "Component'''''''"
sketch "Skizze20" plane through (0, -2, 0) normal (0, -1, 0) x (1, 0, 0)
  line L0 (0, 110) -> (300, 110)
  line L1 (300, 110) -> (300, 112.5)
  line L2 (300, 112.5) -> (0, 112.5)
  line L3 (0, 112.5) -> (0, 110)
  line L4 (0, 112.5) -> (300, 112.5)
  line L5 (300, 112.5) -> (300, 0)
  line L6 (300, 0) -> (0, 0)
  line L7 (0, 0) -> (0, 112.5)
  constraint horizontal L4
  constraint vertical L5
  constraint horizontal L6
  constraint vertical L7
  constraint coincident L2.end L3.start
extrude "Extrusion2''''''" add sketch "Skizze20" along normal blind 2.5 bodies 9 in component "Component'''''''"
component "Component" placed x (1, 0, 0) y (0, 1, 0) z (0, 0, 1) at (0, 0, 0)
component "Component'" placed x (1, 0, 0) y (0, 1, 0) z (0, 0, 1) at (0, 0, 0)
component "Component''" placed x (1, 0, 0) y (0, 1, 0) z (0, 0, 1) at (0, 0, 0)
component "Component'''" placed x (1, 0, 0) y (0, 1, 0) z (0, 0, 1) at (0, 0, 0)
component "Component''''" placed x (1, 0, 0) y (0, 1, 0) z (0, 0, 1) at (0, 0, 0)
component "Component'''''" placed x (1, 0, 0) y (0, 1, 0) z (0, 0, 1) at (0, 0, 0)
component "Component''''''" placed x (1, 0, 0) y (0, 1, 0) z (0, 0, 1) at (0, 0, 0)
component "Component'''''''" placed x (1, 0, 0) y (0, 1, 0) z (0, 0, 1) at (0, 0, 0)
